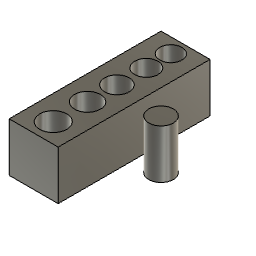
calibrate (Autodesk Fusion 360 design; units mm, degrees)
Autodesk Fusion 360 part; units mm, degrees
sketch "Sketch1" plane through (0, 0, 0) normal (0, 0, 1) x (1, 0, 0)
  circle A0 centre (-5, 22) radius 2.25
  circle A1 centre (-5, 17) radius 2.375
  circle A2 centre (-5, 11) radius 2.5
  circle A3 centre (-5, 5) radius 2.625
  circle A4 centre (-5, -2) radius 2.75
  line L0 (-10, 25) -> (0, 25)
  line L1 (0, 25) -> (0, -6)
  line L2 (0, -6) -> (-10, -6)
  line L3 (-10, -6) -> (-10, 25)
  dimension "d1" = 4.5
  dimension "d2" = 4.75
  dimension "d3" = 5
  dimension "d4" = 5.25
  dimension "d5" = 5.5
  constraint horizontal L0
  constraint vertical L1
  constraint horizontal L2
  constraint vertical L3
  measures "d1" diameter of A0
  measures "d2" diameter of A1
  measures "d3" diameter of A2
  measures "d4" diameter of A3
  measures "d5" diameter of A4
extrude "Extrude1" add sketch "Sketch1" along normal blind 10 makes body 1
sketch "Sketch2" plane through (0, 0, 0) normal (0, 0, 1) x (1, 0, 0)
  circle A0 centre (5, 10) radius 2.5
  dimension "d8" = 5
  measures "d8" diameter of A0
extrude "Extrude2" add sketch "Sketch2" along normal blind 10 separate body makes body 2
